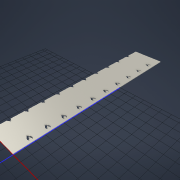
# Autodesk Inventor part: mangal1
Saved by Autodesk Inventor 2022 (Build 260153070, 153G)
## iProperties
Created: 2022-02-16
Part Number: mangal1
Material: Сталь, мягкая
Document SubType Name: Sheet Metal
Designer: kalugin_a
Density: 7.85 g/cm^3
Appearance: Сталь — литейная
Flat Pattern Width: 14.5 cm
Flat Pattern Length: 80 cm
Flat Pattern Area: 1160 cm^2
Sheet Metal Rule: По умолчанию_мм
Sheet Metal Width: 145,000 мм
Sheet Metal Length: 800,000 мм
Sheet Metal Area: 116000,000 мм^2
Author: kalugin_a
Autodesk Inventor part; units mm, degrees
ref_plane "YZ Plane" through (0, 0, 0) normal (1, 0, 0) x (0, 1, 0)
ref_plane "XZ Plane" through (0, 0, 0) normal (0, 1, 0) x (-1, 0, 0)
ref_plane "XY Plane" through (0, 0, 0) normal (0, 0, 1) x (1, 0, 0)
sketch "Эскиз1" plane through (0, 0, 0) normal (0, 1, 0) x (-1, 0, 0)
  line L0 (0, 0) -> (145, 0)
  line L1 (145, 0) -> (145, -800)
  line L2 (145, -800) -> (0, -800)
  line L3 (0, -800) -> (0, 0)
  line L4 (145, -78) -> (145, -68)
  line L5 (10, -70.0424) -> (13.5695, -65.8521) construction
  line L6 (13.5695, -65.8521) -> (19.6532, -69.2354) construction
  spline S0 degree 2 poles (10, -70.0424) (13.5695, -65.8521) (19.6532, -69.2354) knots 1 1 1 2 2 2
  line L7 (19.6532, -69.2354) -> (16.6113, -69.5458) construction
  line L8 (16.6113, -69.5458) -> (16.1768, -71.1909) construction
  spline S1 degree 2 poles (19.6532, -69.2354) (16.6113, -69.5458) (16.1768, -71.1909) knots 1 1 1 2 2 2
  line L9 (16.1768, -71.1909) -> (21.9429, -70.5088) construction
  line L10 (21.9429, -70.5088) -> (25.1161, -74.3258) construction
  spline S2 degree 2 poles (16.1768, -71.1909) (21.9429, -70.5088) (25.1161, -74.3258) knots 1 1 1 2 2 2
  line L11 (25.1161, -74.3258) -> (19.6532, -74.3258) construction
  line L12 (19.6532, -74.3258) -> (16.3941, -82.7685) construction
  line L13 (16.3941, -82.7685) -> (10, -76.4675) construction
  spline S3 degree 3 poles (25.1161, -74.3258) (19.6532, -74.3258) (16.3941, -82.7685) (10, -76.4675) knots 1 1 1 1 2 2 2 2
  line L14 (10, -76.4675) -> (14.7265, -87.0884) construction
  line L15 (14.7265, -87.0884) -> (27.9096, -79.975) construction
  spline S4 degree 2 poles (10, -76.4675) (14.7265, -87.0884) (27.9096, -79.975) knots 1 1 1 2 2 2
  line L16 (27.9096, -79.975) -> (25.6841, -79.5569) construction
  line L17 (25.6841, -79.5569) -> (24.8704, -78.2111) construction
  spline S5 degree 2 poles (27.9096, -79.975) (25.6841, -79.5569) (24.8704, -78.2111) knots 1 1 1 2 2 2
  line L18 (24.8704, -78.2111) -> (33.2958, -78.2111) construction
  line L19 (33.2958, -78.2111) -> (37.0725, -71.1909) construction
  spline S6 degree 2 poles (24.8704, -78.2111) (33.2958, -78.2111) (37.0725, -71.1909) knots 1 1 1 2 2 2
  line L20 (37.0725, -71.1909) -> (27.142, -71.796) construction
  line L21 (27.142, -71.796) -> (26.2598, -61.3671) construction
  line L22 (26.2598, -61.3671) -> (14.3651, -60.2343) construction
  line L23 (14.3651, -60.2343) -> (10, -70.0424) construction
  spline S7 degree 4 poles (37.0725, -71.1909) (27.142, -71.796) (26.2598, -61.3671) (14.3651, -60.2343) (10, -70.0424) knots 1 1 1 1 1 2 2 2 2 2
  line L24 (10, -149.4675) -> (14.7265, -160.0884) construction
  line L25 (16.3941, -155.7685) -> (10, -149.4675) construction
  line L26 (27.9096, -152.975) -> (25.6841, -152.5569) construction
  line L27 (25.6841, -152.5569) -> (24.8704, -151.2111) construction
  spline S8 degree 2 poles (27.9096, -152.975) (25.6841, -152.5569) (24.8704, -151.2111) knots 1 1 1 2 2 2
  line L28 (19.6532, -147.3258) -> (16.3941, -155.7685) construction
  spline S9 degree 2 poles (10, -149.4675) (14.7265, -160.0884) (27.9096, -152.975) knots 1 1 1 2 2 2
  line L29 (14.7265, -160.0884) -> (27.9096, -152.975) construction
  line L30 (25.1161, -147.3258) -> (19.6532, -147.3258) construction
  line L31 (10, -143.0424) -> (13.5695, -138.8521) construction
  line L32 (13.5695, -138.8521) -> (19.6532, -142.2354) construction
  spline S10 degree 2 poles (10, -143.0424) (13.5695, -138.8521) (19.6532, -142.2354) knots 1 1 1 2 2 2
  line L33 (19.6532, -142.2354) -> (16.6113, -142.5458) construction
  line L34 (16.6113, -142.5458) -> (16.1768, -144.1909) construction
  spline S11 degree 2 poles (19.6532, -142.2354) (16.6113, -142.5458) (16.1768, -144.1909) knots 1 1 1 2 2 2
  spline S12 degree 3 poles (25.1161, -147.3258) (19.6532, -147.3258) (16.3941, -155.7685) (10, -149.4675) knots 1 1 1 1 2 2 2 2
  line L35 (16.1768, -144.1909) -> (21.9429, -143.5088) construction
  line L36 (21.9429, -143.5088) -> (25.1161, -147.3258) construction
  spline S13 degree 2 poles (16.1768, -144.1909) (21.9429, -143.5088) (25.1161, -147.3258) knots 1 1 1 2 2 2
  line L37 (24.8704, -151.2111) -> (33.2958, -151.2111) construction
  spline S14 degree 2 poles (24.8704, -151.2111) (33.2958, -151.2111) (37.0725, -144.1909) knots 1 1 1 2 2 2
  line L38 (33.2958, -151.2111) -> (37.0725, -144.1909) construction
  line L39 (27.142, -144.796) -> (26.2598, -134.3671) construction
  line L40 (14.3651, -133.2343) -> (10, -143.0424) construction
  line L41 (26.2598, -134.3671) -> (14.3651, -133.2343) construction
  line L42 (37.0725, -144.1909) -> (27.142, -144.796) construction
  spline S15 degree 4 poles (37.0725, -144.1909) (27.142, -144.796) (26.2598, -134.3671) (14.3651, -133.2343) (10, -143.0424) knots 1 1 1 1 1 2 2 2 2 2
  line L43 (10, -222.4675) -> (14.7265, -233.0884) construction
  line L44 (16.3941, -228.7685) -> (10, -222.4675) construction
  line L45 (27.9096, -225.975) -> (25.6841, -225.5569) construction
  line L46 (25.6841, -225.5569) -> (24.8704, -224.2111) construction
  spline S16 degree 2 poles (27.9096, -225.975) (25.6841, -225.5569) (24.8704, -224.2111) knots 1 1 1 2 2 2
  line L47 (19.6532, -220.3258) -> (16.3941, -228.7685) construction
  spline S17 degree 2 poles (10, -222.4675) (14.7265, -233.0884) (27.9096, -225.975) knots 1 1 1 2 2 2
  line L48 (14.7265, -233.0884) -> (27.9096, -225.975) construction
  line L49 (25.1161, -220.3258) -> (19.6532, -220.3258) construction
  line L50 (10, -216.0424) -> (13.5695, -211.8521) construction
  line L51 (13.5695, -211.8521) -> (19.6532, -215.2354) construction
  spline S18 degree 2 poles (10, -216.0424) (13.5695, -211.8521) (19.6532, -215.2354) knots 1 1 1 2 2 2
  line L52 (19.6532, -215.2354) -> (16.6113, -215.5458) construction
  line L53 (16.6113, -215.5458) -> (16.1768, -217.1909) construction
  spline S19 degree 2 poles (19.6532, -215.2354) (16.6113, -215.5458) (16.1768, -217.1909) knots 1 1 1 2 2 2
  spline S20 degree 3 poles (25.1161, -220.3258) (19.6532, -220.3258) (16.3941, -228.7685) (10, -222.4675) knots 1 1 1 1 2 2 2 2
  line L54 (16.1768, -217.1909) -> (21.9429, -216.5088) construction
  line L55 (21.9429, -216.5088) -> (25.1161, -220.3258) construction
  spline S21 degree 2 poles (16.1768, -217.1909) (21.9429, -216.5088) (25.1161, -220.3258) knots 1 1 1 2 2 2
  line L56 (24.8704, -224.2111) -> (33.2958, -224.2111) construction
  spline S22 degree 2 poles (24.8704, -224.2111) (33.2958, -224.2111) (37.0725, -217.1909) knots 1 1 1 2 2 2
  line L57 (33.2958, -224.2111) -> (37.0725, -217.1909) construction
  line L58 (27.142, -217.796) -> (26.2598, -207.3671) construction
  line L59 (14.3651, -206.2343) -> (10, -216.0424) construction
  line L60 (26.2598, -207.3671) -> (14.3651, -206.2343) construction
  line L61 (37.0725, -217.1909) -> (27.142, -217.796) construction
  spline S23 degree 4 poles (37.0725, -217.1909) (27.142, -217.796) (26.2598, -207.3671) (14.3651, -206.2343) (10, -216.0424) knots 1 1 1 1 1 2 2 2 2 2
  line L62 (10, -295.4675) -> (14.7265, -306.0884) construction
  line L63 (16.3941, -301.7685) -> (10, -295.4675) construction
  line L64 (27.9096, -298.975) -> (25.6841, -298.5569) construction
  line L65 (25.6841, -298.5569) -> (24.8704, -297.2111) construction
  spline S24 degree 2 poles (27.9096, -298.975) (25.6841, -298.5569) (24.8704, -297.2111) knots 1 1 1 2 2 2
  line L66 (19.6532, -293.3258) -> (16.3941, -301.7685) construction
  spline S25 degree 2 poles (10, -295.4675) (14.7265, -306.0884) (27.9096, -298.975) knots 1 1 1 2 2 2
  line L67 (14.7265, -306.0884) -> (27.9096, -298.975) construction
  line L68 (25.1161, -293.3258) -> (19.6532, -293.3258) construction
  line L69 (10, -289.0424) -> (13.5695, -284.8521) construction
  line L70 (13.5695, -284.8521) -> (19.6532, -288.2354) construction
  spline S26 degree 2 poles (10, -289.0424) (13.5695, -284.8521) (19.6532, -288.2354) knots 1 1 1 2 2 2
  line L71 (19.6532, -288.2354) -> (16.6113, -288.5458) construction
  line L72 (16.6113, -288.5458) -> (16.1768, -290.1909) construction
  spline S27 degree 2 poles (19.6532, -288.2354) (16.6113, -288.5458) (16.1768, -290.1909) knots 1 1 1 2 2 2
  spline S28 degree 3 poles (25.1161, -293.3258) (19.6532, -293.3258) (16.3941, -301.7685) (10, -295.4675) knots 1 1 1 1 2 2 2 2
  line L73 (16.1768, -290.1909) -> (21.9429, -289.5088) construction
  line L74 (21.9429, -289.5088) -> (25.1161, -293.3258) construction
  spline S29 degree 2 poles (16.1768, -290.1909) (21.9429, -289.5088) (25.1161, -293.3258) knots 1 1 1 2 2 2
  line L75 (24.8704, -297.2111) -> (33.2958, -297.2111) construction
  spline S30 degree 2 poles (24.8704, -297.2111) (33.2958, -297.2111) (37.0725, -290.1909) knots 1 1 1 2 2 2
  line L76 (33.2958, -297.2111) -> (37.0725, -290.1909) construction
  line L77 (27.142, -290.796) -> (26.2598, -280.3671) construction
  line L78 (14.3651, -279.2343) -> (10, -289.0424) construction
  line L79 (26.2598, -280.3671) -> (14.3651, -279.2343) construction
  line L80 (37.0725, -290.1909) -> (27.142, -290.796) construction
  spline S31 degree 4 poles (37.0725, -290.1909) (27.142, -290.796) (26.2598, -280.3671) (14.3651, -279.2343) (10, -289.0424) knots 1 1 1 1 1 2 2 2 2 2
  line L81 (10, -368.4675) -> (14.7265, -379.0884) construction
  line L82 (16.3941, -374.7685) -> (10, -368.4675) construction
  line L83 (27.9096, -371.975) -> (25.6841, -371.5569) construction
  line L84 (25.6841, -371.5569) -> (24.8704, -370.2111) construction
  spline S32 degree 2 poles (27.9096, -371.975) (25.6841, -371.5569) (24.8704, -370.2111) knots 1 1 1 2 2 2
  line L85 (19.6532, -366.3258) -> (16.3941, -374.7685) construction
  spline S33 degree 2 poles (10, -368.4675) (14.7265, -379.0884) (27.9096, -371.975) knots 1 1 1 2 2 2
  line L86 (14.7265, -379.0884) -> (27.9096, -371.975) construction
  line L87 (25.1161, -366.3258) -> (19.6532, -366.3258) construction
  line L88 (10, -362.0424) -> (13.5695, -357.8521) construction
  line L89 (13.5695, -357.8521) -> (19.6532, -361.2354) construction
  spline S34 degree 2 poles (10, -362.0424) (13.5695, -357.8521) (19.6532, -361.2354) knots 1 1 1 2 2 2
  line L90 (19.6532, -361.2354) -> (16.6113, -361.5458) construction
  line L91 (16.6113, -361.5458) -> (16.1768, -363.1909) construction
  spline S35 degree 2 poles (19.6532, -361.2354) (16.6113, -361.5458) (16.1768, -363.1909) knots 1 1 1 2 2 2
  spline S36 degree 3 poles (25.1161, -366.3258) (19.6532, -366.3258) (16.3941, -374.7685) (10, -368.4675) knots 1 1 1 1 2 2 2 2
  line L92 (16.1768, -363.1909) -> (21.9429, -362.5088) construction
  line L93 (21.9429, -362.5088) -> (25.1161, -366.3258) construction
  spline S37 degree 2 poles (16.1768, -363.1909) (21.9429, -362.5088) (25.1161, -366.3258) knots 1 1 1 2 2 2
  line L94 (24.8704, -370.2111) -> (33.2958, -370.2111) construction
  spline S38 degree 2 poles (24.8704, -370.2111) (33.2958, -370.2111) (37.0725, -363.1909) knots 1 1 1 2 2 2
  line L95 (33.2958, -370.2111) -> (37.0725, -363.1909) construction
  line L96 (27.142, -363.796) -> (26.2598, -353.3671) construction
  line L97 (14.3651, -352.2343) -> (10, -362.0424) construction
  line L98 (26.2598, -353.3671) -> (14.3651, -352.2343) construction
  line L99 (37.0725, -363.1909) -> (27.142, -363.796) construction
  spline S39 degree 4 poles (37.0725, -363.1909) (27.142, -363.796) (26.2598, -353.3671) (14.3651, -352.2343) (10, -362.0424) knots 1 1 1 1 1 2 2 2 2 2
  line L100 (10, -441.4675) -> (14.7265, -452.0884) construction
  line L101 (16.3941, -447.7685) -> (10, -441.4675) construction
  line L102 (27.9096, -444.975) -> (25.6841, -444.5569) construction
  line L103 (25.6841, -444.5569) -> (24.8704, -443.2111) construction
  spline S40 degree 2 poles (27.9096, -444.975) (25.6841, -444.5569) (24.8704, -443.2111) knots 1 1 1 2 2 2
  line L104 (19.6532, -439.3258) -> (16.3941, -447.7685) construction
  spline S41 degree 2 poles (10, -441.4675) (14.7265, -452.0884) (27.9096, -444.975) knots 1 1 1 2 2 2
  line L105 (14.7265, -452.0884) -> (27.9096, -444.975) construction
  line L106 (25.1161, -439.3258) -> (19.6532, -439.3258) construction
  line L107 (10, -435.0424) -> (13.5695, -430.8521) construction
  line L108 (13.5695, -430.8521) -> (19.6532, -434.2354) construction
  spline S42 degree 2 poles (10, -435.0424) (13.5695, -430.8521) (19.6532, -434.2354) knots 1 1 1 2 2 2
  line L109 (19.6532, -434.2354) -> (16.6113, -434.5458) construction
  line L110 (16.6113, -434.5458) -> (16.1768, -436.1909) construction
  spline S43 degree 2 poles (19.6532, -434.2354) (16.6113, -434.5458) (16.1768, -436.1909) knots 1 1 1 2 2 2
  spline S44 degree 3 poles (25.1161, -439.3258) (19.6532, -439.3258) (16.3941, -447.7685) (10, -441.4675) knots 1 1 1 1 2 2 2 2
  line L111 (16.1768, -436.1909) -> (21.9429, -435.5088) construction
  line L112 (21.9429, -435.5088) -> (25.1161, -439.3258) construction
  spline S45 degree 2 poles (16.1768, -436.1909) (21.9429, -435.5088) (25.1161, -439.3258) knots 1 1 1 2 2 2
  line L113 (24.8704, -443.2111) -> (33.2958, -443.2111) construction
  spline S46 degree 2 poles (24.8704, -443.2111) (33.2958, -443.2111) (37.0725, -436.1909) knots 1 1 1 2 2 2
  line L114 (33.2958, -443.2111) -> (37.0725, -436.1909) construction
  line L115 (27.142, -436.796) -> (26.2598, -426.3671) construction
  line L116 (14.3651, -425.2343) -> (10, -435.0424) construction
  line L117 (26.2598, -426.3671) -> (14.3651, -425.2343) construction
  line L118 (37.0725, -436.1909) -> (27.142, -436.796) construction
  spline S47 degree 4 poles (37.0725, -436.1909) (27.142, -436.796) (26.2598, -426.3671) (14.3651, -425.2343) (10, -435.0424) knots 1 1 1 1 1 2 2 2 2 2
  line L119 (10, -514.4675) -> (14.7265, -525.0884) construction
  line L120 (16.3941, -520.7685) -> (10, -514.4675) construction
  line L121 (27.9096, -517.975) -> (25.6841, -517.5569) construction
  line L122 (25.6841, -517.5569) -> (24.8704, -516.2111) construction
  spline S48 degree 2 poles (27.9096, -517.975) (25.6841, -517.5569) (24.8704, -516.2111) knots 1 1 1 2 2 2
  line L123 (19.6532, -512.3258) -> (16.3941, -520.7685) construction
  spline S49 degree 2 poles (10, -514.4675) (14.7265, -525.0884) (27.9096, -517.975) knots 1 1 1 2 2 2
  line L124 (14.7265, -525.0884) -> (27.9096, -517.975) construction
  line L125 (25.1161, -512.3258) -> (19.6532, -512.3258) construction
  line L126 (10, -508.0424) -> (13.5695, -503.8521) construction
  line L127 (13.5695, -503.8521) -> (19.6532, -507.2354) construction
  spline S50 degree 2 poles (10, -508.0424) (13.5695, -503.8521) (19.6532, -507.2354) knots 1 1 1 2 2 2
  line L128 (19.6532, -507.2354) -> (16.6113, -507.5458) construction
  line L129 (16.6113, -507.5458) -> (16.1768, -509.1909) construction
  spline S51 degree 2 poles (19.6532, -507.2354) (16.6113, -507.5458) (16.1768, -509.1909) knots 1 1 1 2 2 2
  spline S52 degree 3 poles (25.1161, -512.3258) (19.6532, -512.3258) (16.3941, -520.7685) (10, -514.4675) knots 1 1 1 1 2 2 2 2
  line L130 (16.1768, -509.1909) -> (21.9429, -508.5088) construction
  line L131 (21.9429, -508.5088) -> (25.1161, -512.3258) construction
  spline S53 degree 2 poles (16.1768, -509.1909) (21.9429, -508.5088) (25.1161, -512.3258) knots 1 1 1 2 2 2
  line L132 (24.8704, -516.2111) -> (33.2958, -516.2111) construction
  spline S54 degree 2 poles (24.8704, -516.2111) (33.2958, -516.2111) (37.0725, -509.1909) knots 1 1 1 2 2 2
  line L133 (33.2958, -516.2111) -> (37.0725, -509.1909) construction
  line L134 (27.142, -509.796) -> (26.2598, -499.3671) construction
  line L135 (14.3651, -498.2343) -> (10, -508.0424) construction
  line L136 (26.2598, -499.3671) -> (14.3651, -498.2343) construction
  line L137 (37.0725, -509.1909) -> (27.142, -509.796) construction
  spline S55 degree 4 poles (37.0725, -509.1909) (27.142, -509.796) (26.2598, -499.3671) (14.3651, -498.2343) (10, -508.0424) knots 1 1 1 1 1 2 2 2 2 2
  line L138 (10, -587.4675) -> (14.7265, -598.0884) construction
  line L139 (16.3941, -593.7685) -> (10, -587.4675) construction
  line L140 (27.9096, -590.975) -> (25.6841, -590.5569) construction
  line L141 (25.6841, -590.5569) -> (24.8704, -589.2111) construction
  spline S56 degree 2 poles (27.9096, -590.975) (25.6841, -590.5569) (24.8704, -589.2111) knots 1 1 1 2 2 2
  line L142 (19.6532, -585.3258) -> (16.3941, -593.7685) construction
  spline S57 degree 2 poles (10, -587.4675) (14.7265, -598.0884) (27.9096, -590.975) knots 1 1 1 2 2 2
  line L143 (14.7265, -598.0884) -> (27.9096, -590.975) construction
  line L144 (25.1161, -585.3258) -> (19.6532, -585.3258) construction
  line L145 (10, -581.0424) -> (13.5695, -576.8521) construction
  line L146 (13.5695, -576.8521) -> (19.6532, -580.2354) construction
  spline S58 degree 2 poles (10, -581.0424) (13.5695, -576.8521) (19.6532, -580.2354) knots 1 1 1 2 2 2
  line L147 (19.6532, -580.2354) -> (16.6113, -580.5458) construction
  line L148 (16.6113, -580.5458) -> (16.1768, -582.1909) construction
  spline S59 degree 2 poles (19.6532, -580.2354) (16.6113, -580.5458) (16.1768, -582.1909) knots 1 1 1 2 2 2
  spline S60 degree 3 poles (25.1161, -585.3258) (19.6532, -585.3258) (16.3941, -593.7685) (10, -587.4675) knots 1 1 1 1 2 2 2 2
  line L149 (16.1768, -582.1909) -> (21.9429, -581.5088) construction
  line L150 (21.9429, -581.5088) -> (25.1161, -585.3258) construction
  spline S61 degree 2 poles (16.1768, -582.1909) (21.9429, -581.5088) (25.1161, -585.3258) knots 1 1 1 2 2 2
  line L151 (24.8704, -589.2111) -> (33.2958, -589.2111) construction
  spline S62 degree 2 poles (24.8704, -589.2111) (33.2958, -589.2111) (37.0725, -582.1909) knots 1 1 1 2 2 2
  line L152 (33.2958, -589.2111) -> (37.0725, -582.1909) construction
  line L153 (27.142, -582.796) -> (26.2598, -572.3671) construction
  line L154 (14.3651, -571.2343) -> (10, -581.0424) construction
  line L155 (26.2598, -572.3671) -> (14.3651, -571.2343) construction
  line L156 (37.0725, -582.1909) -> (27.142, -582.796) construction
  spline S63 degree 4 poles (37.0725, -582.1909) (27.142, -582.796) (26.2598, -572.3671) (14.3651, -571.2343) (10, -581.0424) knots 1 1 1 1 1 2 2 2 2 2
  line L157 (10, -660.4675) -> (14.7265, -671.0884) construction
  line L158 (16.3941, -666.7685) -> (10, -660.4675) construction
  line L159 (27.9096, -663.975) -> (25.6841, -663.5569) construction
  line L160 (25.6841, -663.5569) -> (24.8704, -662.2111) construction
  spline S64 degree 2 poles (27.9096, -663.975) (25.6841, -663.5569) (24.8704, -662.2111) knots 1 1 1 2 2 2
  line L161 (19.6532, -658.3258) -> (16.3941, -666.7685) construction
  spline S65 degree 2 poles (10, -660.4675) (14.7265, -671.0884) (27.9096, -663.975) knots 1 1 1 2 2 2
  line L162 (14.7265, -671.0884) -> (27.9096, -663.975) construction
  line L163 (25.1161, -658.3258) -> (19.6532, -658.3258) construction
  line L164 (10, -654.0424) -> (13.5695, -649.8521) construction
  line L165 (13.5695, -649.8521) -> (19.6532, -653.2354) construction
  spline S66 degree 2 poles (10, -654.0424) (13.5695, -649.8521) (19.6532, -653.2354) knots 1 1 1 2 2 2
  line L166 (19.6532, -653.2354) -> (16.6113, -653.5458) construction
  line L167 (16.6113, -653.5458) -> (16.1768, -655.1909) construction
  spline S67 degree 2 poles (19.6532, -653.2354) (16.6113, -653.5458) (16.1768, -655.1909) knots 1 1 1 2 2 2
  spline S68 degree 3 poles (25.1161, -658.3258) (19.6532, -658.3258) (16.3941, -666.7685) (10, -660.4675) knots 1 1 1 1 2 2 2 2
  line L168 (16.1768, -655.1909) -> (21.9429, -654.5088) construction
  line L169 (21.9429, -654.5088) -> (25.1161, -658.3258) construction
  spline S69 degree 2 poles (16.1768, -655.1909) (21.9429, -654.5088) (25.1161, -658.3258) knots 1 1 1 2 2 2
  line L170 (24.8704, -662.2111) -> (33.2958, -662.2111) construction
  spline S70 degree 2 poles (24.8704, -662.2111) (33.2958, -662.2111) (37.0725, -655.1909) knots 1 1 1 2 2 2
  line L171 (33.2958, -662.2111) -> (37.0725, -655.1909) construction
  line L172 (27.142, -655.796) -> (26.2598, -645.3671) construction
  line L173 (14.3651, -644.2343) -> (10, -654.0424) construction
  line L174 (26.2598, -645.3671) -> (14.3651, -644.2343) construction
  line L175 (37.0725, -655.1909) -> (27.142, -655.796) construction
  spline S71 degree 4 poles (37.0725, -655.1909) (27.142, -655.796) (26.2598, -645.3671) (14.3651, -644.2343) (10, -654.0424) knots 1 1 1 1 1 2 2 2 2 2
  line L176 (10, -733.4675) -> (14.7265, -744.0884) construction
  line L177 (16.3941, -739.7685) -> (10, -733.4675) construction
  line L178 (27.9096, -736.975) -> (25.6841, -736.5569) construction
  line L179 (25.6841, -736.5569) -> (24.8704, -735.2111) construction
  spline S72 degree 2 poles (27.9096, -736.975) (25.6841, -736.5569) (24.8704, -735.2111) knots 1 1 1 2 2 2
  line L180 (19.6532, -731.3258) -> (16.3941, -739.7685) construction
  spline S73 degree 2 poles (10, -733.4675) (14.7265, -744.0884) (27.9096, -736.975) knots 1 1 1 2 2 2
  line L181 (14.7265, -744.0884) -> (27.9096, -736.975) construction
  line L182 (25.1161, -731.3258) -> (19.6532, -731.3258) construction
  line L183 (10, -727.0424) -> (13.5695, -722.8521) construction
  line L184 (13.5695, -722.8521) -> (19.6532, -726.2354) construction
  spline S74 degree 2 poles (10, -727.0424) (13.5695, -722.8521) (19.6532, -726.2354) knots 1 1 1 2 2 2
  line L185 (19.6532, -726.2354) -> (16.6113, -726.5458) construction
  line L186 (16.6113, -726.5458) -> (16.1768, -728.1909) construction
  spline S75 degree 2 poles (19.6532, -726.2354) (16.6113, -726.5458) (16.1768, -728.1909) knots 1 1 1 2 2 2
  spline S76 degree 3 poles (25.1161, -731.3258) (19.6532, -731.3258) (16.3941, -739.7685) (10, -733.4675) knots 1 1 1 1 2 2 2 2
  line L187 (16.1768, -728.1909) -> (21.9429, -727.5088) construction
  line L188 (21.9429, -727.5088) -> (25.1161, -731.3258) construction
  spline S77 degree 2 poles (16.1768, -728.1909) (21.9429, -727.5088) (25.1161, -731.3258) knots 1 1 1 2 2 2
  line L189 (24.8704, -735.2111) -> (33.2958, -735.2111) construction
  spline S78 degree 2 poles (24.8704, -735.2111) (33.2958, -735.2111) (37.0725, -728.1909) knots 1 1 1 2 2 2
  line L190 (33.2958, -735.2111) -> (37.0725, -728.1909) construction
  line L191 (27.142, -728.796) -> (26.2598, -718.3671) construction
  line L192 (14.3651, -717.2343) -> (10, -727.0424) construction
  line L193 (26.2598, -718.3671) -> (14.3651, -717.2343) construction
  line L194 (37.0725, -728.1909) -> (27.142, -728.796) construction
  spline S79 degree 4 poles (37.0725, -728.1909) (27.142, -728.796) (26.2598, -718.3671) (14.3651, -717.2343) (10, -727.0424) knots 1 1 1 1 1 2 2 2 2 2
  circle A0 centre (145, -73) radius 7.5
  line L195 (137.9897, -70.5) -> (132.9897, -70.5)
  line L196 (132.9897, -70.5) -> (132.9897, -75.5)
  line L197 (132.9897, -75.5) -> (137.9897, -75.5)
  line L198 (137.9897, -75.5) -> (137.9897, -70.5)
  line L199 (137.9897, -70.5) -> (132.9897, -75.5) construction
  line L200 (132.9897, -70.5) -> (137.9897, -75.5) construction
  circle A1 centre (145, -146) radius 7.5
  line L201 (137.9897, -143.5) -> (132.9897, -143.5)
  line L202 (132.9897, -143.5) -> (132.9897, -148.5)
  line L203 (132.9897, -148.5) -> (137.9897, -148.5)
  circle A2 centre (145, -219) radius 7.5
  line L204 (137.9897, -216.5) -> (132.9897, -216.5)
  line L205 (132.9897, -216.5) -> (132.9897, -221.5)
  line L206 (132.9897, -221.5) -> (137.9897, -221.5)
  circle A3 centre (145, -292) radius 7.5
  line L207 (137.9897, -289.5) -> (132.9897, -289.5)
  line L208 (132.9897, -289.5) -> (132.9897, -294.5)
  line L209 (132.9897, -294.5) -> (137.9897, -294.5)
  circle A4 centre (145, -365) radius 7.5
  line L210 (137.9897, -362.5) -> (132.9897, -362.5)
  line L211 (132.9897, -362.5) -> (132.9897, -367.5)
  line L212 (132.9897, -367.5) -> (137.9897, -367.5)
  circle A5 centre (145, -438) radius 7.5
  line L213 (137.9897, -435.5) -> (132.9897, -435.5)
  line L214 (132.9897, -435.5) -> (132.9897, -440.5)
  line L215 (132.9897, -440.5) -> (137.9897, -440.5)
  circle A6 centre (145, -511) radius 7.5
  line L216 (137.9897, -508.5) -> (132.9897, -508.5)
  line L217 (132.9897, -508.5) -> (132.9897, -513.5)
  line L218 (132.9897, -513.5) -> (137.9897, -513.5)
  circle A7 centre (145, -584) radius 7.5
  line L219 (137.9897, -581.5) -> (132.9897, -581.5)
  line L220 (132.9897, -581.5) -> (132.9897, -586.5)
  line L221 (132.9897, -586.5) -> (137.9897, -586.5)
  circle A8 centre (145, -657) radius 7.5
  line L222 (137.9897, -654.5) -> (132.9897, -654.5)
  line L223 (132.9897, -654.5) -> (132.9897, -659.5)
  line L224 (132.9897, -659.5) -> (137.9897, -659.5)
  circle A9 centre (145, -730) radius 7.5
  line L225 (137.9897, -727.5) -> (132.9897, -727.5)
  line L226 (132.9897, -727.5) -> (132.9897, -732.5)
  line L227 (132.9897, -732.5) -> (137.9897, -732.5)
  point P0 (135, -73)
  point P1 (137.5, -73)
  point P2 (137.9289, -70.5)
  point P3 (137.9025, -75.5)
  point P4 (135.4897, -73)
  point P5 (137.5, -146)
  point P6 (137.9289, -143.5)
  point P7 (137.5, -219)
  point P8 (137.9289, -216.5)
  point P9 (137.5, -292)
  point P10 (137.9289, -289.5)
  point P11 (137.5, -365)
  point P12 (137.9289, -362.5)
  point P13 (137.5, -438)
  point P14 (137.9289, -435.5)
  point P15 (137.5, -511)
  point P16 (137.9289, -508.5)
  point P17 (137.5, -584)
  point P18 (137.9289, -581.5)
  point P19 (137.5, -657)
  point P20 (137.9289, -654.5)
  point P21 (137.5, -730)
  point P22 (137.9289, -727.5)
  point P23 (145, -737.5)
  point P24 (137.9289, -732.5)
  point P25 (137.9289, -727.5)
  point P26 (145, -722.5)
  point P27 (145, -664.5)
  point P28 (137.9289, -659.5)
  point P29 (137.9289, -654.5)
  point P30 (145, -649.5)
  point P31 (145, -591.5)
  point P32 (137.9289, -586.5)
  point P33 (137.9289, -581.5)
  point P34 (145, -576.5)
  point P35 (145, -518.5)
  point P36 (137.9289, -513.5)
  point P37 (137.9289, -508.5)
  point P38 (145, -503.5)
  point P39 (145, -445.5)
  point P40 (137.9289, -440.5)
  point P41 (137.9289, -435.5)
  point P42 (145, -430.5)
  point P43 (145, -372.5)
  point P44 (137.9289, -367.5)
  point P45 (137.9289, -362.5)
  point P46 (145, -357.5)
  point P47 (145, -299.5)
  point P48 (137.9289, -294.5)
  point P49 (137.9289, -289.5)
  point P50 (145, -284.5)
  point P51 (145, -226.5)
  point P52 (137.9289, -221.5)
  point P53 (137.9289, -216.5)
  point P54 (145, -211.5)
  point P55 (145, -153.5)
  point P56 (137.9289, -148.5)
  point P57 (137.9289, -143.5)
  point P58 (145, -138.5)
  point P59 (145, -80.5)
  point P60 (137.9289, -75.5)
  point P61 (137.9289, -70.5)
  point P62 (145, -65.5)
  dimension "d0" = 145
  dimension "d1" = 800
  dimension "d102" = 10
  dimension "d105" = 73
  dimension "d110" = 15
  dimension "d124" = 5
  dimension "d125" = 5
  dimension "d128" = 73
  constraints: 74 end point, 74 vertical, 63 vertical alignment, 21 parallel, 20 point on circle, 10 centre point, 9 collinear, 9 equal radius, 3 horizontal, 2 midpoint, 1 perpendicular, 586 other
  measures "d0" distance of L2.start L2.end
  measures "d1" distance of L0.end L2.start
  measures "d102" distance from line of L3 L13.end
  measures "d105" distance of L14.end L24.end
  measures "d110" diameter of A0
  measures "d124" distance of L196.end L197.end
  measures "d125" distance of L195.end L196.end
  measures "d128" distance of A0.centre A1.centre
extrude "Выдавливание3" add sketch "Эскиз1" along normal blind 3 contours L0 L1 A0 L195 L196 L197 A1 L201 L202 L203 A2 L204 L205 L206 A3 L207 L208 L209 A4 L210 L211 L212 A5 L213 L214 L215 A6 L216 L217 L218 A7 L219 L220 L221 A8 L222 L223 L224 A9 L225 L226 L227 L2 L3
equation "\"Радиус_гибки\" = Толщина"
equation "\"Ширина_просечки\" = Толщина"
equation "\"Радиус_перехода\" = Радиус_гибки"
equation "\"Радиус_Якоби\" = Радиус_гибки"
equation "\"Размер_зазора\" = Толщина"
equation "\"Толщина\" = 3"
